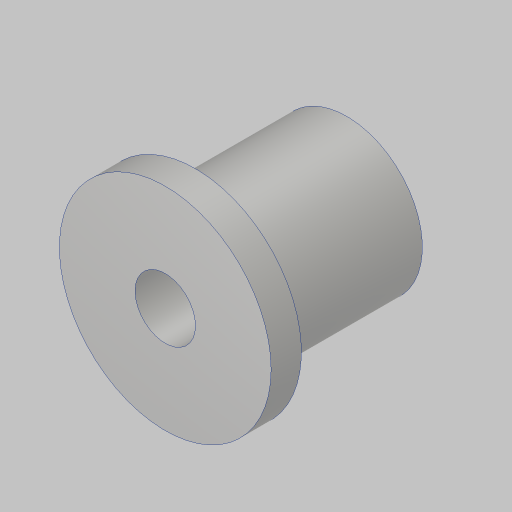
# Autodesk Inventor part: AR-013
Saved by Autodesk Inventor 2023.5 (Build 275446000, 446)
## iProperties
Created: 2025-01-31
Part Number: AR-013
Material: Aluminum 6061
Document SubType Name: Modeling
Designer: slick
Density: 2.7 g/cm^3
Appearance: Aluminum - Flat
Author: slick
Autodesk Inventor part; units mm, degrees
ref_plane "YZ Plane" through (0, 0, 0) normal (1, 0, 0) x (0, 1, 0)
ref_plane "XZ Plane" through (0, 0, 0) normal (0, 1, 0) x (-1, 0, 0)
ref_plane "XY Plane" through (0, 0, 0) normal (0, 0, 1) x (1, 0, 0)
sketch "Sketch1" plane through (0, 0, 0) normal (0, 0, 1) x (1, 0, 0)
  circle A0 centre (0, 0) radius 11.1125
  dimension "d0" = 22.225
  constraints: 1 centre point, 1 coincident
  measures "d0" diameter of A0
extrude "Extrusion1" add sketch "Sketch1" along normal mid plane 19.05
sketch "Sketch3" plane through (0, 0, -9.525) normal (0, 0, -1) x (-1, 0, 0)
  circle A0 centre (0, 0) radius 11.1125 projected
  circle A1 centre (0, 0) radius 7.9375
  dimension "d6" = 15.875
  constraints: 1 centre point, 1 coincident
  measures "d6" diameter of A1
extrude "Extrusion3" cut sketch "Sketch3" against normal blind 15.875
sketch "Sketch5" plane through (0, 0, -9.525) normal (0, 0, -1) x (-1, 0, 0)
  circle A0 centre (0, 0) radius 7.9375 construction
  constraints: 1 coincident
hole "Hole2" at (0, 0, -9.525) direction (0, 0, 1) diameter 6.35 end through all
body "Solid1"
